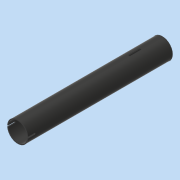
# Autodesk Inventor part: PrimaryHullLexanTube_01
Saved by Autodesk Inventor 2017.3 (Build 213256000, 256)
## iProperties
Created: 2016-09-09
Part Number: PrimaryHullLexanTube_01
Material: Polycarbonate, Clear
Document SubType Name: Modeling
Designer: techn
Density: 1.2 g/cm^3
Appearance: Smooth - Black
Mass: 835.743 g
Surface Area: 4410.94 cm^2
Volume: 696.452 cm^3
Author: techn
Autodesk Inventor part; units mm, degrees
ref_plane "YZ Plane" through (0, 0, 0) normal (1, 0, 0) x (0, 1, 0)
ref_plane "XY Plane" through (0, 0, 0) normal (0, 0, 1) x (1, 0, 0)
sketch "Sketch1" plane through (0, 0, 0) normal (0, 0, 1) x (1, 0, 0)
  circle A0 centre (0, 0) radius 50.8
  circle A1 centre (0, 0) radius 47.625
  dimension "d0" = 101.6
  dimension "d1" = 95.25
  constraints: 2 centre point, 2 coincident
  measures "d0" diameter of A0
  measures "d1" diameter of A1
extrude "Extrusion1" add sketch "Sketch1" along normal blind 711.2
ref_plane "Work Plane1" through (0, 50.8, 0) normal (0, 1, 0) x (-1, 0, 0)
sketch "Sketch5" plane through (0, 0, 0) normal (1, 0, 0) x (0, 1, 0)
  line L0 (50.8, 711.2) -> (-50.8, 711.2) construction
  line L1 (-50.8, 0) -> (50.8, 0) construction
  line L2 (3.175, 711.2) -> (-3.175, 711.2)
  line L3 (-3.175, 711.2) -> (-3.175, 678.7388)
  line L4 (3.175, 678.7388) -> (3.175, 711.2)
  arc A0 (-3.175, 678.7388) -> (3.175, 678.7388) centre (0, 678.7388) ccw
  line L5 (0, 769.9295) -> (0, 0) construction
  dimension "d16" = 3.175
  dimension "d17" = 32.4612
  constraints: 8 end point, 2 point on circle, 2 point on line, 2 tangent, 1 centre point, 1 horizontal, 1 parallel, 1 perpendicular, 1 vertical
  measures "d16" radius of A0
  measures "d17" distance from line of L0 A0.centre
extrude "Extrusion4" cut sketch "Sketch5" along normal through all both and the other way through all
sketch "Sketch6" plane through (0, 0, 0) normal (0, 1, 0) x (-1, 0, 0)
  line L0 (4.7625, 203.2) -> (4.7625, 165.1)
  line L1 (-4.7625, 203.2) -> (-4.7625, 165.1)
  arc A0 (4.7625, 203.2) -> (-4.7625, 203.2) centre (0, 203.2) ccw
  arc A1 (-4.7625, 165.1) -> (4.7625, 165.1) centre (0, 165.1) ccw
  point P0 (0, 0)
  dimension "d20" = 203.2
  dimension "d21" = 165.1
  dimension "d22" = 9.525
  constraints: 4 end point, 4 point on circle, 4 tangent, 2 centre point, 2 vertical, 1 vertical alignment
  measures "d20" distance of point (0, 0) A0.centre
  measures "d21" distance of point (0, 0) A1.centre
  measures "d22" distance between parallel lines of L0 L1
extrude "Extrusion5" cut sketch "Sketch6" against normal through all
sketch "Sketch7" plane through (0, 50.8, 0) normal (0, 1, 0) x (-1, 0, 0)
  line L0 (4.7625, 161.925) -> (4.7625, 107.95)
  line L1 (-4.7625, 107.95) -> (-4.7625, 161.925)
  arc A0 (-4.7625, 107.95) -> (4.7625, 107.95) centre (0, 107.95) ccw
  arc A1 (4.7625, 161.925) -> (-4.7625, 161.925) centre (0, 161.925) ccw
  line L2 (-50.8, 0) -> (50.8, 0) projected
  point P0 (0, 0)
  dimension "d25" = 107.95
  dimension "d26" = 161.925
  dimension "d27" = 9.525
  constraints: 4 end point, 4 point on circle, 4 tangent, 2 centre point, 2 vertical, 1 vertical alignment
  measures "d25" distance from line of A0.centre L2
  measures "d26" distance from line of L2 A1.centre
  measures "d27" distance between parallel lines of L1 L0
extrude "Extrusion6" cut sketch "Sketch7" against normal blind 25.4
body "Solid1"
